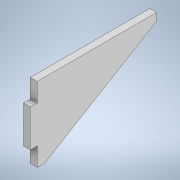
# Autodesk Inventor part: Bracket
Saved by Autodesk Inventor 2020 (Build 240168000, 168)
## iProperties
Created: 2019-12-27
Part Number: Bracket
Material: Générique
Document SubType Name: Modeling
Designer: damien
Density: 1 g/cm^3
Appearance: Par défaut
Author: damien
Autodesk Inventor part; units mm, degrees
ref_plane "YZ Plane" through (0, 0, 0) normal (1, 0, 0) x (0, 1, 0)
ref_plane "XZ Plane" through (0, 0, 0) normal (0, 1, 0) x (-1, 0, 0)
ref_plane "XY Plane" through (0, 0, 0) normal (0, 0, 1) x (1, 0, 0)
sketch "Esquisse1" plane through (0, 0, 0) normal (1, 0, 0) x (0, 1, 0)
  line L0 (0, 0) -> (-200, 0)
  line L1 (-200, 0) -> (-200, -20)
  line L2 (-200, -20) -> (-20, -320)
  line L3 (-20, -320) -> (0, -320)
  line L4 (0, -320) -> (0, 0)
  dimension "d0" = 200
  dimension "d1" = 20
  dimension "d2" = 20
  dimension "d3" = 320
  constraints: 10 end point, 2 perpendicular, 1 horizontal, 1 parallel
  measures "d0" distance of L0.start L0.end
  measures "d1" distance of L2.end L3.end
  measures "d2" distance of L0.end L1.end
  measures "d3" distance of L3.end L0.start
extrude "Extrusion1" add sketch "Esquisse1" along normal blind 18.55
sketch "Esquisse2" plane through (18.55, 0, 0) normal (1, 0, 0) x (0, 0, -1)
  line L0 (0, 0) -> (0, -200) projected
  line L1 (0, -50.1) -> (-18.55, -50.1)
  line L2 (-18.55, -50.1) -> (-18.55, -149.9)
  line L3 (-18.55, -149.9) -> (0, -149.9)
  line L4 (0, -149.9) -> (0, -50.1)
  line L5 (320, 0) -> (0, 0) projected
  point P0 (0, -149.9)
  dimension "d6" = 18.55
  dimension "d7" = 50.1
  dimension "d8" = 99.8
  constraints: 8 end point, 2 parallel, 1 horizontal, 1 perpendicular, 1 point on line
  measures "d6" distance of L1.start L1.end
  measures "d7" distance between parallel lines of L5 L1
  measures "d8" distance of L1.end L2.end
extrude "Extrusion2" add sketch "Esquisse2" against normal blind 18.55
sketch "Esquisse3" plane through (18.55, 0, 0) normal (1, 0, 0) x (0, 0, -1)
  circle A0 centre (-1.1314, -48.9686) radius 1.6
  line L0 (-1.1314, -48.9686) -> (0, -50.1) construction
  line L1 (0, -50.1) -> (-18.55, -50.1) projected
  circle A1 centre (-1.1314, -151.0314) radius 1.6
  point P0 (0, 0)
  point P1 (0, -149.9)
  dimension "d12" = 3.2
  dimension "d11" = 45
  constraints: 2 end point, 1 vertical alignment, 6 other
  measures "d11" angle of L1 L0
extrude "Extrusion3" cut sketch "Esquisse3" against normal blind 18.55
